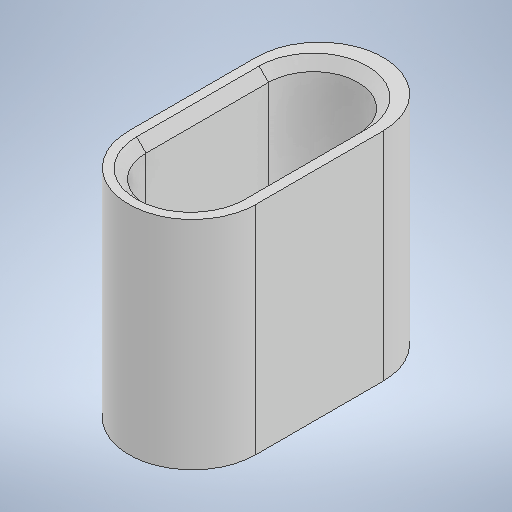
# Autodesk Inventor part: motor-tuningpeg
Saved by Autodesk Inventor 2025.2 (Build 292293000, 293)
## iProperties
Created: 2025-03-05
Part Number: motor-tuningpeg
Material: Generic
Document SubType Name: Modeling
Designer: 3lin2
Density: 1 g/cm^3
Appearance: Default
Author: 3lin2
Autodesk Inventor part; units mm, degrees
ref_plane "YZ Plane" through (0, 0, 0) normal (1, 0, 0) x (0, 1, 0)
ref_plane "XZ Plane" through (0, 0, 0) normal (0, 1, 0) x (-1, 0, 0)
ref_plane "XY Plane" through (0, 0, 0) normal (0, 0, 1) x (1, 0, 0)
sketch "Sketch1" plane through (0, 0, 0) normal (0, 1, 0) x (-1, 0, 0)
  line L0 (-0.0336, 5.4315) -> (-0.0336, -7.5685) construction
  line L1 (-0.0384, 6.7095) -> (-0.0384, -6.7905) construction
  line L2 (-6.7884, 6.7095) -> (-6.7884, -6.7905)
  line L3 (6.7116, -6.7905) -> (6.7116, 6.7095)
  arc A0 (6.7116, 6.7095) -> (-6.7884, 6.7095) centre (-0.0384, 6.7095) ccw
  arc A1 (-6.7884, -6.7905) -> (6.7116, -6.7905) centre (-0.0384, -6.7905) ccw
  point P0 (0, 0)
  point P1 (-0.0384, -0.0405)
  point P2 (-0.0384, -13.5405)
  point P3 (-0.0384, 13.4595)
  dimension "d4" = 13.5
  dimension "d5" = 27
  constraints: 12 end point, 6 point on circle, 4 tangent, 2 centre point, 2 vertical, 1 midpoint, 1 parallel
  measures "d4" diameter of A1
  measures "d5" distance of point (-0.038, -13.54) point (-0.038, 13.46)
extrude "Extrusion1" add sketch "Sketch1" along normal blind 23
sketch "Sketch4" plane through (0, 23, 0) normal (0, 1, 0) x (1, 0, 0)
  line L0 (0, 6.1571) -> (0, -6.8429) construction
  line L1 (-4.75, 6.1571) -> (-4.75, -6.8429)
  line L2 (4.75, -6.8429) -> (4.75, 6.1571)
  arc A0 (4.75, 6.1571) -> (-4.75, 6.1571) centre (0, 6.1571) ccw
  arc A1 (-4.75, -6.8429) -> (4.75, -6.8429) centre (0, -6.8429) ccw
  point P0 (0, 0)
  point P1 (0, -0.3429)
  point P2 (0, -11.5929)
  point P3 (0, 10.9071)
  point P4 (4.75, -0.3429)
  point P5 (-4.75, -0.3429)
  dimension "d11" = 22.5
  dimension "d12" = 9.5
  constraints: 8 end point, 6 point on circle, 4 tangent, 3 midpoint, 2 centre point, 1 parallel, 1 vertical
  measures "d11" distance of point (0, -11.593) point (0, 10.907)
  measures "d12" distance of point (4.75, -0.343) point (-4.75, -0.343)
extrude "Extrusion2" cut sketch "Sketch4" against normal blind 18
sketch "Sketch5" plane through (0, 0, 0) normal (0, -1, 0) x (1, 0, 0)
  circle A0 centre (0, 0) radius 1.55
  line L0 (1.1402, -1.05) -> (-1.1402, -1.05)
  point P0 (0, -1.05)
  dimension "d15" = 3.1
  dimension "d16" = 1.05
  constraints: 2 end point, 2 point on circle, 1 centre point, 1 coincident, 1 horizontal, 1 midpoint
  measures "d15" diameter of A0
  measures "d16" distance of A0.centre point (0, -1.05)
extrude "Extrusion3" cut sketch "Sketch5" against normal blind 18 contours A0 L0 picked at (0.3868, -0.1503)
chamfer "Chamfer1" distance 1 angle 45 4 edges at (-4.75, 23, 0.3429) (0, 23, -10.9071) (4.75, 23, 0.3429) (0, 23, 11.5929)
body "Solid1"
